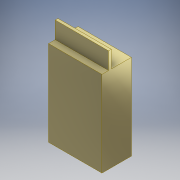
# Autodesk Inventor part: Module_CO2Sensor-T6713
Saved by Autodesk Inventor 2018 (Build 220112000, 112)
## iProperties
Created: 2018-07-29
Part Number: Module_CO2Sensor-T6713
Material: ABS Plastic
Document SubType Name: Modeling
Designer: Bradley
Density: 1.06 g/cm^3
Appearance: Gold - Metal
Author: Bradley
Autodesk Inventor part; units mm, degrees
ref_plane "YZ Plane" through (0, 0, 0) normal (1, 0, 0) x (0, 1, 0)
ref_plane "XZ Plane" through (0, 0, 0) normal (0, 1, 0) x (-1, 0, 0)
ref_plane "XY Plane" through (0, 0, 0) normal (0, 0, 1) x (1, 0, 0)
sketch "Sketch1" plane through (0, 0, 0) normal (0, 1, 0) x (-1, 0, 0)
  line L0 (-7.8, 14.985) -> (7.8, 14.985)
  line L1 (7.8, 14.985) -> (7.8, -14.985)
  line L2 (7.8, -14.985) -> (-7.8, -14.985)
  line L3 (-7.8, -14.985) -> (-7.8, 14.985)
  line L4 (-7.8, 14.985) -> (7.8, -14.985) construction
  line L5 (7.8, 14.985) -> (-7.8, -14.985) construction
  point P0 (0, 0)
  dimension "d0" = 15.6
  dimension "d1" = 29.97
  constraints: 12 end point, 2 midpoint, 2 parallel, 1 horizontal, 1 perpendicular
  measures "d0" distance of L1.end L2.end
  measures "d1" distance of L0.end L1.end
extrude "Extrusion1" add sketch "Sketch1" along normal mid plane 0.8
sketch "Sketch2" plane through (0, 0.4, 0) normal (0, 1, 0) x (1, 0, 0)
  line L0 (-7.8, -14.985) -> (7.8, -14.985) projected
  line L1 (7.8, -14.985) -> (7.8, 14.985) projected
  line L2 (7.8, 14.985) -> (-7.8, 14.985) projected
  line L3 (-7.8, 14.985) -> (-7.8, -14.985) projected
  line L4 (7.8, 14.985) -> (-7.8, 14.985) projected
  line L5 (7.8, -14.985) -> (7.8, 14.985) projected
  line L6 (-7.8, 14.985) -> (7.8, 14.985)
  line L7 (7.8, 14.985) -> (7.8, -10.015)
  line L8 (7.8, -10.015) -> (-7.8, -10.015)
  line L9 (-7.8, -10.015) -> (-7.8, 14.985)
  point P0 (0, 0)
  dimension "d4" = 25
  constraints: 8 end point, 2 parallel, 1 horizontal, 1 perpendicular, 1 point on line
  measures "d4" distance of L6.end L7.end
extrude "Extrusion2" add sketch "Sketch2" along normal blind 5.86 and the other way blind 2.75 contours L3 L2 L1 L8
body "Solid1"
